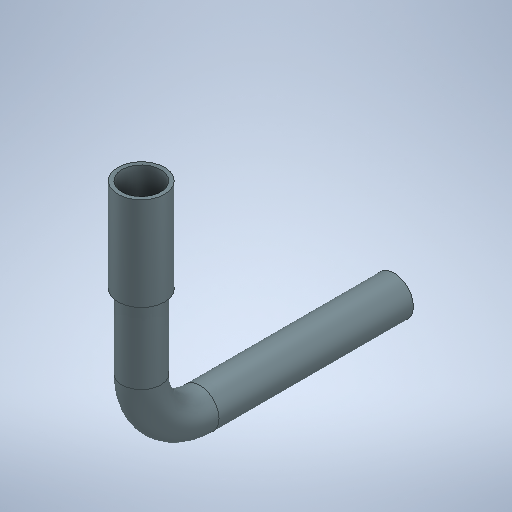
# Autodesk Inventor part: 161
Saved by Autodesk Inventor 2025.1 (Build 291241000, 241)
## iProperties
Created: 2024-08-03
Part Number: 161
Material: Iron, Cast
Document SubType Name: Modeling
Designer: ffogue
Density: 7.15 g/cm^3
Appearance: Lead
Author: ffogue
Autodesk Inventor part; units mm, degrees
ref_plane "YZ Plane" through (0, 0, 0) normal (1, 0, 0) x (0, 1, 0)
ref_plane "XZ Plane" through (0, 0, 0) normal (0, 1, 0) x (-1, 0, 0)
ref_plane "XY Plane" through (0, 0, 0) normal (0, 0, 1) x (1, 0, 0)
sketch "Sketch1" plane through (0, 0, 0) normal (0, 0, 1) x (1, 0, 0)
  circle A0 centre (0, 0) radius 2.5
  dimension "d0" = 5
  constraints: 1 centre point, 1 coincident
  measures "d0" diameter of A0
sketch "Sketch2" plane through (0, 0, 0) normal (1, 0, 0) x (0, 1, 0)
  line L0 (0, 0) -> (0, -15.5)
  line L1 (7.5, -23) -> (32.5, -23)
  arc A0 (0, -15.5) -> (7.5, -23) centre (7.5, -15.5) ccw
  point P0 (0, -23)
  dimension "d1" = 23
  dimension "d2" = 7.5
  dimension "d3" = 25
  constraints: 4 end point, 2 point on circle, 2 point on line, 2 tangent, 1 centre point, 1 perpendicular, 1 vertical
  measures "d1" distance of L0.start point (0, -23)
  measures "d2" radius of A0
  measures "d3" horizontal distance of L1.end A0.centre
sweep "Sweep1" add profiles "Sketch1" path "Sketch2"
sketch "Sketch3" plane through (0, 0, 0) normal (0, 0, 1) x (1, 0, 0)
  circle A0 centre (0, 0) radius 3
  dimension "d6" = 6
  constraints: 1 centre point, 1 coincident
  measures "d6" diameter of A0
extrude "Extrusion1" add sketch "Sketch3" along normal mid plane 12
shell "Shell1" thickness 0.5 removed faces 2 at (-0.5351, 1.0949, 6) at (-0.2146, 32.5, -22.3381)
body "Solid1"
